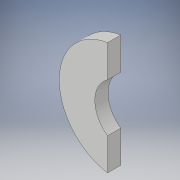
# Autodesk Inventor part: ContrapesoGrande2
Saved by Autodesk Inventor 2019 (Build 230136000, 136)
## iProperties
Created: 2019-06-29
Part Number: ContrapesoGrande2
Material: Generic
Document SubType Name: Modeling
Designer: usuario
Density: 1 g/cm^3
Appearance: Default
Author: usuario
Autodesk Inventor part; units mm, degrees
ref_plane "YZ Plane" through (0, 0, 0) normal (1, 0, 0) x (0, 1, 0)
ref_plane "XZ Plane" through (0, 0, 0) normal (0, 1, 0) x (-1, 0, 0)
ref_plane "XY Plane" through (0, 0, 0) normal (0, 0, 1) x (1, 0, 0)
sketch "Sketch1" plane through (0, 0, 0) normal (0, 0, 1) x (1, 0, 0)
  arc A0 (-5, 32.1131) -> (-5, -32.1131) centre (0, 0) ccw
  arc A1 (-5, 13.7954) -> (-5, -13.7954) centre (4.5, 0) ccw
  line L0 (-5, -13.7954) -> (-5, -32.1131)
  line L1 (-5, 13.7954) -> (-5, 32.1131)
  arc A2 (-5, 13.7954) -> (-5, -13.7954) centre (4.5, 0) ccw
  point P0 (3.7885, 24.6247)
  constraints: 6 point on circle, 4 end point, 3 centre point, 2 vertical, 1 coincident
extrude "Extrusion1" add sketch "Sketch1" along normal blind 7.5
body "Solid1"
